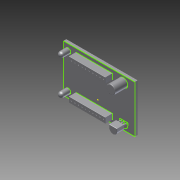
# Autodesk Inventor part: Adafruit xbee adapter
Saved by Autodesk Inventor 2012 (Build 160160000, 160)
## iProperties
Created: 2012-03-02
Part Number: Adafruit xbee adapter
Material: Default
Document SubType Name: Modeling
Designer: Lauszus
Density: 1 g/cm^3
Author: Lauszus
Autodesk Inventor part; units mm, degrees
ref_plane "YZ Plane" through (0, 0, 0) normal (1, 0, 0) x (0, 1, 0)
ref_plane "XZ Plane" through (0, 0, 0) normal (0, 1, 0) x (-1, 0, 0)
ref_plane "XY Plane" through (0, 0, 0) normal (0, 0, 1) x (1, 0, 0)
sketch "Sketch1" plane through (0, 0, 0) normal (0, 0, 1) x (1, 0, 0)
  line L0 (20.6647, -7.5943) -> (-19.3353, -7.5943)
  line L1 (-19.3353, -7.5943) -> (-19.3353, 18.9057)
  line L2 (-19.3353, 18.9057) -> (20.6647, 18.9057)
  line L3 (20.6647, 18.9057) -> (20.6647, -7.5943)
  line L4 (-12.3353, 16.9057) -> (8.1647, 16.9057)
  line L5 (8.1647, 16.9057) -> (8.1647, 13.9057)
  line L6 (8.1647, 13.9057) -> (-12.3353, 13.9057)
  line L7 (-12.3353, 13.9057) -> (-12.3353, 16.9057)
  circle A0 centre (-16.8353, -4.0943) radius 1.5
  circle A1 centre (-16.8353, 15.4057) radius 1.5
  circle A2 centre (14.1647, 15.4057) radius 2.5
  line L8 (16.6647, -4.3443) -> (16.6647, -2.8443)
  line L9 (16.6647, -2.8443) -> (12.1647, -2.8443)
  line L10 (12.1647, -2.8443) -> (12.1647, -4.3443)
  arc A3 (12.1647, -4.3443) -> (16.6647, -4.3443) centre (14.4147, -4.3443) ccw
  line L11 (12.7075, -3.3443) -> (13.2075, -3.3443)
  line L12 (13.2075, -3.3443) -> (13.2075, -3.8443)
  line L13 (13.2075, -3.8443) -> (12.7075, -3.8443)
  line L14 (12.7075, -3.8443) -> (12.7075, -3.3443)
  line L15 (14.2075, -3.3443) -> (14.7075, -3.3443)
  line L16 (14.7075, -3.3443) -> (14.7075, -3.8443)
  line L17 (14.7075, -3.8443) -> (14.2075, -3.8443)
  line L18 (14.2075, -3.8443) -> (14.2075, -3.3443)
  line L19 (15.7075, -3.3443) -> (16.2075, -3.3443)
  line L20 (16.2075, -3.3443) -> (16.2075, -3.8443)
  line L21 (16.2075, -3.8443) -> (15.7075, -3.8443)
  line L22 (15.7075, -3.8443) -> (15.7075, -3.3443)
  circle A4 centre (-10.9431, 15.4057) radius 0.3
  circle A5 centre (-8.9431, 15.4057) radius 0.3
  circle A6 centre (-6.9431, 15.4057) radius 0.3
  circle A7 centre (-4.9431, 15.4057) radius 0.3
  circle A8 centre (-2.9431, 15.4057) radius 0.3
  circle A9 centre (-0.9431, 15.4057) radius 0.3
  circle A10 centre (3.0569, 15.4057) radius 0.3
  circle A11 centre (1.0569, 15.4057) radius 0.3
  circle A12 centre (5.0569, 15.4057) radius 0.3
  circle A13 centre (7.0569, 15.4057) radius 0.3
  line L23 (-12.3353, -2.5943) -> (8.1647, -2.5943)
  line L24 (8.1647, -2.5943) -> (8.1647, -5.5943)
  line L25 (8.1647, -5.5943) -> (-12.3353, -5.5943)
  line L26 (-12.3353, -5.5943) -> (-12.3353, -2.5943)
  circle A14 centre (-10.9431, -4.0943) radius 0.3
  circle A15 centre (-8.9431, -4.0943) radius 0.3
  circle A16 centre (-4.9431, -4.0943) radius 0.3
  circle A17 centre (-6.9431, -4.0943) radius 0.3
  circle A18 centre (-0.9431, -4.0943) radius 0.3
  circle A19 centre (-2.9431, -4.0943) radius 0.3
  circle A20 centre (1.0569, -4.0943) radius 0.3
  circle A21 centre (3.0569, -4.0943) radius 0.3
  circle A22 centre (7.0569, -4.0943) radius 0.3
  circle A23 centre (5.0569, -4.0943) radius 0.3
  point P0 (0, 0)
  dimension "d0" = 40
  dimension "d1" = 26.5
  dimension "d3" = 20.5
  dimension "d4" = 3
  dimension "d6" = 7
  dimension "d8" = 3
  dimension "d9" = 3
  dimension "d10" = 1
  dimension "d11" = 1
  dimension "d12" = 5
  dimension "d13" = 4
  dimension "d14" = 1
  dimension "d23" = 1.5
  dimension "d24" = 4.5
  dimension "d28" = 1
  dimension "d29" = 4
  dimension "d33" = 0.5
  dimension "d34" = 0.5
  dimension "d35" = 0.5
  dimension "d36" = 0.5
  dimension "d37" = 0.5
  dimension "d38" = 0.5
  dimension "d39" = 1
  dimension "d40" = 1
  dimension "d41" = 0.5
  dimension "d42" = 0.5
  dimension "d43" = 0.5
  dimension "d44" = 0.4572
  dimension "d50" = 0.6
  dimension "d51" = 1.0922
  dimension "d52" = 0.6
  dimension "d53" = 2
  dimension "d54" = 1.5
  dimension "d55" = 2
  dimension "d56" = 2
  dimension "d57" = 1.5
  dimension "d58" = 2
  dimension "d60" = 0.6
  dimension "d61" = 0.6
  dimension "d62" = 2
  dimension "d63" = 2
  dimension "d65" = 1.5
  dimension "d66" = 1.5
  dimension "d67" = 0.6
  dimension "d68" = 0.6
  dimension "d69" = 2
  dimension "d70" = 0.6
  dimension "d71" = 0.6
  dimension "d72" = 2
  dimension "d73" = 2
  dimension "d74" = 2
  dimension "d75" = 1.5
  dimension "d76" = 1.5
  dimension "d77" = 1.5
  dimension "d78" = 1.5
  dimension "d79" = 0.6
  dimension "d80" = 0.6
  dimension "d81" = 2
  dimension "d82" = 2
  dimension "d83" = 1.5
  dimension "d84" = 1.5
  dimension "d85" = 20.5
  dimension "d86" = 3
  dimension "d87" = 0.6
  constraints: 54 end point, 24 centre point, 13 parallel, 6 horizontal, 6 perpendicular, 2 point on circle, 2 tangent
  measures "d0" distance of L1.end L2.end
  measures "d1" distance of L0.end L1.end
  measures "d3" distance of L4.start L4.end
  measures "d4" distance of L6.end L4.start
  measures "d6" distance between parallel lines of L1 L7
  measures "d8" diameter of A1
  measures "d9" diameter of A0
  measures "d10" distance edge to line of A0 L1
  measures "d11" distance edge to line of A1 L1
  measures "d12" diameter of A2
  measures "d13" distance edge to line of A2 L3
  measures "d14" distance edge to line of A2 L2
  measures "d23" distance of L8.start L8.end
  measures "d24" distance of L8.end L9.end
  measures "d28" distance edge to line of A3 L0
  measures "d29" distance between parallel lines of L3 L8
  measures "d33" distance of L19.start L19.end
  measures "d34" distance of L19.end L20.end
  measures "d35" distance of L15.end L16.end
  measures "d36" distance of L16.end L17.end
  measures "d37" distance of L11.end L12.end
  measures "d38" distance of L12.end L13.end
  measures "d39" distance between parallel lines of L16 L22
  measures "d40" distance between parallel lines of L12 L18
  measures "d41" distance between parallel lines of L9 L19
  measures "d42" distance between parallel lines of L9 L15
  measures "d43" distance between parallel lines of L9 L11
  measures "d44" distance between parallel lines of L8 L20
  measures "d50" diameter of A4
  measures "d51" distance edge to line of A4 L7
  measures "d52" diameter of A5
  measures "d53" distance between centres of A5 A4
  measures "d54" distance from line of L6 A5.centre
  measures "d55" distance between parallel lines of L2 L4
  measures "d56" distance edge to line of A1 L2
  measures "d57" distance from line of L6 A4.centre
  measures "d58" distance edge to line of A0 L0
  measures "d60" diameter of A6
  measures "d61" diameter of A7
  measures "d62" distance between centres of A7 A6
  measures "d63" distance of A5.centre A6.centre
  measures "d65" distance from line of A7.centre L6
  measures "d66" distance from line of L6 A6.centre
  measures "d67" diameter of A8
  measures "d68" diameter of A9
  measures "d69" distance between centres of A9 A8
  measures "d70" diameter of A11
  measures "d71" diameter of A10
  measures "d72" distance between centres of A10 A11
  measures "d73" distance of A9.centre A11.centre
  measures "d74" distance of A7.centre A8.centre
  measures "d75" distance from line of L6 A8.centre
  measures "d76" distance from line of L6 A9.centre
  measures "d77" distance from line of L6 A11.centre
  measures "d78" distance from line of L6 A10.centre
  measures "d79" diameter of A12
  measures "d80" diameter of A13
  measures "d81" distance between centres of A13 A12
  measures "d82" distance of A10.centre A12.centre
  measures "d83" distance from line of L6 A12.centre
  measures "d84" distance from line of L6 A13.centre
  measures "d85" distance of L23.start L23.end
  measures "d86" distance of L25.end L23.start
  measures "d87" diameter of A14
extrude "Extrusion1" add sketch "Sketch1" against normal blind 1.6 contours L0 L1 L2 L3 | L4 L5 L6 L7 | A0 | A1 | A2 | A3 L10 L9 L8 | L11 L12 L13 L14 | L15 L16 L17 L18 | L19 L20 L21 L22 | A4 | A5 | A6 | A7 | A8 | A9 | A10 | A11 | A12 | A13 | L23 L24 L25 L26 | A14 | A15 | A16 | A17 | A18 | A19 | A20 | A21 | A22 | A23
extrude "Extrusion2" add sketch "Sketch1" along normal blind 7 contours A2
extrude "Extrusion3" add sketch "Sketch1" along normal blind 5 contours A0 | A1
fillet "Fillet1" radius 1.4986 2 edges at (-18.3353, -4.0943, 5) (-18.3353, 15.4057, 5)
fillet "Fillet2" radius 0.254 1 edges at (11.6647, 15.4057, 7)
extrude "Extrusion5" add sketch "Sketch1" along normal blind 2 contours L11 L12 L13 L14 | L15 L16 L17 L18 | L19 L20 L21 L22
ref_plane "Work Plane1" through (0, 0, 1) normal (0, 0, 1) x (1, 0, 0)
sketch "Sketch2" plane through (0, 0, 2) normal (0, 0, 1) x (1, 0, 0)
  line L0 (14.7075, -3.8443) -> (14.2075, -3.8443) projected
  line L1 (12.1708, -2.8384) -> (16.6562, -2.8384)
  line L2 (16.6562, -2.8384) -> (16.6562, -4.3569)
  line L3 (12.1708, -4.3569) -> (12.1708, -2.8384)
  arc A0 (12.1708, -4.3569) -> (16.6562, -4.3569) centre (14.4135, -4.3569) ccw
  point P0 (0, 0)
  constraints: 6 end point, 2 parallel, 2 point on circle, 2 tangent, 1 centre point, 1 perpendicular
extrude "Extrusion6" add sketch "Sketch2" along normal blind 4
fillet "Fillet4" radius 0.254 4 edges at (14.4135, -2.8384, 6) (12.1708, -3.5977, 6) (16.6562, -3.5977, 6) (14.4135, -6.5996, 6)
extrude "Extrusion7" add sketch "Sketch1" along normal blind 4 contours L4 L5 L6 L7 | L23 L24 L25 L26
fillet "Fillet5" radius 0.127 8 edges at (-2.0853, 16.9057, 4) (-12.3353, 15.4057, 4) (-2.0853, 13.9057, 4) (8.1647, 15.4057, 4) (8.1647, -4.0943, 4) (-2.0853, -2.5943, 4) (-12.3353, -4.0943, 4) (-2.0853, -5.5943, 4)
body "Solid1"
